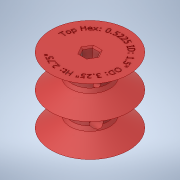
# Autodesk Inventor part: spoolV07
Saved by Autodesk Inventor 2020.2 (Build 242310000, 310)
## iProperties
Created: 2019-02-25
Part Number: spoolV07
Material: PC/ABS Plastic
Document SubType Name: Modeling
Designer: steele
Density: 0.357273 g/cm^3
Appearance: Smooth - Red
holeForString: 0.200 in
stringDiameter: 0.120 in
clearanceForString: 0.080 in
clearanceForHexShaft: 0.023 in
hexDiameter: 0.523 in
supportChannels: 0.150 in
spoolInteriorDiameter: 1.500 in
spoolInteriroRadius: 0.750 in
spoolExteriorDiameter: 3.250 in
spoolExteriorRadius: 1.625 in
spoolFiletRadius: 0.075 in
holeCenter: 0.575 in
hexHoleChamfer: 0.063 in
stringHoleCenterFromHexShaft: 0.361 in
textCircleDiameter: 2.438 in
textHeight: 0.240 in
textDepth: 0.050 in
stringHoleChamfer: 0.188 in
spoolTotalHeight: 3.000 in
spaceHeight: 0.250 in
spacerDiameter: 0.950 in
spoolHeightWithoutSpacer: 2.750 in
Author: steele
Autodesk Inventor part; units mm, degrees
(part 1 of 2)
ref_plane "XZ Plane" through (0, 0, 0) normal (0, 1, 0) x (-1, 0, 0)
ref_plane "XY Plane" through (0, 0, 0) normal (0, 0, 1) x (1, 0, 0)
sketch "Sketch15" plane through (0, 0, 0) normal (0, 0, 1) x (1, 0, 0)
  line L0 (41.275, 0) -> (41.275, 69.85) construction
  line L1 (0, 0) -> (41.275, 0)
  line L2 (0, 69.85) -> (41.275, 69.85)
  line L3 (19.05, 0) -> (19.05, 69.85) construction
  line L4 (0, 69.85) -> (0, 0)
  line L5 (19.05, 17.4625) -> (41.275, 17.4625) construction
  line L6 (41.275, 0) -> (19.05, 12.8316)
  line L7 (41.275, 34.925) -> (19.05, 22.0934)
  line L8 (19.05, 22.0934) -> (41.275, 22.0934) construction
  line L9 (19.05, 22.0934) -> (19.05, 12.8316)
  line L10 (41.275, 34.925) -> (19.05, 47.7566)
  line L11 (19.05, 47.7566) -> (19.05, 57.0184)
  line L12 (19.05, 57.0184) -> (41.275, 69.85)
  line L13 (41.275, 34.925) -> (19.05, 34.925) construction
  line L14 (19.05, 57.0184) -> (41.275, 57.0184) construction
  dimension "d85" = 41.275
  dimension "d86" = 69.85
  dimension "d87" = 19.05
  dimension "d88" = 41.275
  dimension "d89" = 34.925
  dimension "centerLineForSpool" = 17.4625
  dimension "d93" = 30
  dimension "d94" = 30
  dimension "d95" = 30
  dimension "d96" = 30
  constraints: 30 end point, 10 point on line, 3 horizontal, 2 midpoint, 2 perpendicular, 1 collinear, 1 parallel, 1 vertical
  measures "d85" distance from line of L1.start L0
  measures "d86" distance of L0.start L0.end
  measures "d87" distance from line of L3 L1.start
  measures "d88" distance of L2.start L0.end
  measures "d89" distance from line of L7.start L1
  measures "centerLineForSpool" distance from line of L5.start L1
  measures "d93" angle of L6 L1
  measures "d94" angle of L7 L8
  measures "d95" angle of L10 L13
  measures "d96" angle of L12 L14
revolve "Revolution2" add sketch "Sketch15" angle 360 about axis through (0, 69.85, 0) along (0, -1, 0)
sketch "Sketch16" plane through (0, 0, 0) normal (0, -1, 0) x (1, 0, 0)
  line L0 (-7.6623, 0) -> (-3.8312, 6.6357)
  line L1 (-3.8312, 6.6357) -> (3.8312, 6.6357)
  line L2 (3.8312, 6.6357) -> (7.6623, 0)
  line L3 (7.6623, 0) -> (3.8312, -6.6358)
  line L4 (3.8312, -6.6358) -> (-3.8312, -6.6358)
  line L5 (-3.8312, -6.6358) -> (-7.6623, 0)
  point P0 (0, 0)
  point P1 (0, 0)
  dimension "d103" = 13.2715
  constraints: 12 end point, 1 coincident, 1 horizontal, 13 other
  measures "d103" distance between parallel lines of L1 L4
extrude "Extrusion11" cut sketch "Sketch16" against normal through all
sketch "Sketch17" plane through (0, 0, 0) normal (1, 0, 0) x (0, 1, 0)
  circle A0 centre (52.3875, 9.1757) radius 2.54
  circle A1 centre (17.4625, 9.1757) radius 2.54
  line L0 (0, 41.275) -> (0, -41.275) projected
  line L1 (69.85, 41.275) -> (69.85, -41.275) projected
  line L2 (0, 6.6357) -> (69.85, 6.6357) projected
  point P0 (0, 0)
  dimension "d110" = 17.4625
  dimension "d111" = 17.4625
  dimension "d112" = 5.08
  constraints: 2 centre point, 2 tangent, 1 equal radius
  measures "d110" distance from line of A1.centre L0
  measures "d111" distance from line of A0.centre L1
  measures "d112" diameter of A0
extrude "Extrusion13" cut sketch "Sketch17" along normal through all both and the other way through all
ref_plane "Work Plane4" through (-19.05, 0, 0) normal (1, 0, 0) x (0, 1, 0)
sketch "Sketch22" plane through (-19.05, 0, 0) normal (1, 0, 0) x (0, 1, 0)
  spline S0 degree 8 poles (54.9275, 9.1757) (54.9275, 9.4517) (54.8932, 9.7212) (54.8275, 9.9804) (54.7331, 10.2261) (54.613, 10.4557) (54.4698, 10.6669) (54.3066, 10.858) (53.9519, 11.191) (53.76, 11.336) (53.5529, 11.4599) (53.3333, 11.5609) (53.1042, 11.6378) (52.8683, 11.6896) (52.6284, 11.7157) (52.1061, 11.7157) (51.8268, 11.6801) (51.5538, 11.6098) (51.2914, 11.5059) (51.0437, 11.37) (50.815, 11.2041) (50.6094, 11.0111) (50.2522, 10.5794) (50.097, 10.3366) (49.9708, 10.0693) (49.879, 9.7817) (49.8257, 9.479) (49.8146, 9.1672) (49.848, 8.8531) (50.0407, 8.1024) (50.2409, 7.6991) (50.5126, 7.3483) (50.8412, 7.0608) (51.2104, 6.8444) (51.6031, 6.703) (52.001, 6.6357) (52.6651, 6.6357) (52.944, 6.6704) (53.2202, 6.7403) (53.4892, 6.8459) (53.7465, 6.9871) (53.9869, 7.1637) (54.2051, 7.3748) (54.5207, 7.7816) (54.6337, 7.9584) (54.7307, 8.1474) (54.8096, 8.3459) (54.869, 8.5511) (54.9083, 8.76) (54.9275, 8.9692) (54.9275, 9.1757) knots 0 0 0 0 0 0 0 0 0 0.129052 0.129052 0.129052 0.129052 0.129052 0.129052 0.129052 0.253777 0.253777 0.253777 0.253777 0.253777 0.253777 0.253777 0.399469 0.399469 0.399469 0.399469 0.399469 0.399469 0.399469 0.544533 0.544533 0.544533 0.544533 0.544533 0.544533 0.544533 0.751894 0.751894 0.751894 0.751894 0.751894 0.751894 0.751894 0.900801 0.900801 0.900801 0.900801 0.900801 0.900801 0.900801 1 1 1 1 1 1 1 1 1 projected
  circle A0 centre (52.3875, 9.1757) radius 4.7625
  circle A1 centre (52.3875, 9.1757) radius 2.54 construction
  line L0 (52.3875, 6.6357) -> (69.85, 6.6357) construction
  line L1 (69.85, 41.275) -> (69.85, -41.275) construction
  point P0 (0, 0)
  dimension "d121" = 17.4625
  dimension "d122" = 5.08
  dimension "d125" = 9.525
  constraints: 2 centre point, 1 concentric, 1 tangent, 1 vertical alignment
  measures "d121" distance from line of A1.centre L1
  measures "d122" diameter of A1
  measures "d125" diameter of A0
extrude "Extrusion16" cut sketch "Sketch22" along normal blind 11.1125
ref_plane "Work Plane5" through (19.05, 0, 0) normal (1, 0, 0) x (0, 1, 0)
sketch "Sketch23" plane through (19.05, 0, 0) normal (1, 0, 0) x (0, 1, 0)
  line L0 (17.4625, 6.6357) -> (52.3875, 6.6357) projected
  circle A0 centre (17.4625, 9.1757) radius 2.54 construction
  line L1 (0, 41.275) -> (0, -41.275) projected
  circle A1 centre (17.4625, 9.1757) radius 4.7625
  point P0 (0, 0)
  dimension "d127" = 5.08
  dimension "d128" = 17.4625
  dimension "d129" = 9.525
  constraints: 2 centre point, 1 coincident, 1 tangent
  measures "d127" diameter of A0
  measures "d128" distance from line of A0.centre L1
  measures "d129" diameter of A1
extrude "Extrusion17" cut sketch "Sketch23" against normal blind 11.1125
chamfer "Chamfer10" distance 1.5875 angle 45 12 edges at (0, 69.85, -6.6358) (5.7467, 69.85, -3.3179) (5.7467, 69.85, 3.3179) (0, 69.85, 6.6357) (-5.7467, 69.85, 3.3179) (-5.7467, 69.85, -3.3179) (-5.7467, 0, -3.3179) (-5.7467, 0, 3.3179) (0, 0, 6.6357) (5.7467, 0, 3.3179) (5.7467, 0, -3.3179) (0, 0, -6.6358)
chamfer "Chamfer12" distance 2.3813 angle 45 8 edges at (-4.1302, 57.0184, -18.5969) (5.3604, 57.0184, 18.2803) (-4.1302, 47.7566, -18.5969) (5.3604, 47.7566, 18.2803) (-18.2803, 22.0934, -5.3604) (18.5969, 22.0934, 4.1302) (18.5969, 12.8316, 4.1302) (-18.2803, 12.8316, -5.3604)
ref_plane "Work Plane6" through (0, 38.1, 0) normal (0, -1, 0) x (1, 0, 0)
sketch "Sketch24" plane through (0, 69.85, 0) normal (0, 1, 0) x (1, 0, 0)
  circle A0 centre (0, 0) radius 28.575 construction
  line L0 (-28.5166, 1.8645) -> (-33.4283, 2.2505)
  line L1 (-33.4283, 2.2505) -> (-33.5752, 0.3816)
  line L2 (-33.5752, 0.3816) -> (-34.2343, 0.4334)
  line L3 (-34.2343, 0.4334) -> (-33.8823, 4.9117)
  line L4 (-33.8823, 4.9117) -> (-33.2232, 4.8599)
  line L5 (-33.2232, 4.8599) -> (-33.3701, 2.9909)
  line L6 (-33.3701, 2.9909) -> (-28.4584, 2.6048)
  line L7 (-28.4584, 2.6048) -> (-28.5166, 1.8645)
  spline S0 degree 2 poles (-29.4394, 8.8077) (-28.4076, 8.5664) (-27.5153, 7.3113) (-27.7091, 6.4823) knots 0 0 0 1 2 2 2
  spline S1 degree 2 poles (-27.7091, 6.4823) (-27.9081, 5.6313) (-29.2957, 4.9281) (-30.2922, 5.1611) knots 0 0 0 1 2 2 2
  spline S2 degree 2 poles (-30.2922, 5.1611) (-31.3152, 5.4003) (-32.2133, 6.6707) (-32.0215, 7.4908) knots 0 0 0 1 2 2 2
  spline S3 degree 2 poles (-32.0215, 7.4908) (-31.8276, 8.3198) (-30.4668, 9.0479) (-29.4394, 8.8077) knots 0 0 0 1 2 2 2
  spline S4 degree 2 poles (-29.6055, 8.0978) (-30.3991, 8.2834) (-31.3059, 7.8862) (-31.4306, 7.3527) knots 0 0 0 1 2 2 2
  spline S5 degree 2 poles (-31.4306, 7.3527) (-31.5554, 6.8191) (-30.9199, 6.0566) (-30.1262, 5.871) knots 0 0 0 1 2 2 2
  spline S6 degree 2 poles (-30.1262, 5.871) (-29.3546, 5.6906) (-28.4247, 6.087) (-28.3, 6.6205) knots 0 0 0 1 2 2 2
  spline S7 degree 2 poles (-28.3, 6.6205) (-28.1762, 7.1496) (-28.8206, 7.9142) (-29.6055, 8.0978) knots 0 0 0 1 2 2 2
  spline S8 degree 2 poles (-27.9258, 13.0947) (-26.9489, 12.7082) (-26.1634, 11.3211) (-26.445, 10.6095) knots 0 0 0 1 2 2 2
  spline S9 degree 2 poles (-26.445, 10.6095) (-26.5599, 10.3189) (-26.8713, 9.9259) (-27.1019, 9.7493) knots 0 0 0 1 2 2 2
  line L8 (-27.1019, 9.7493) -> (-25.4681, 9.1029)
  line L9 (-25.4681, 9.1029) -> (-25.728, 8.446)
  line L10 (-25.728, 8.446) -> (-31.063, 10.5569)
  line L11 (-31.063, 10.5569) -> (-30.8031, 11.2138)
  line L12 (-30.8031, 11.2138) -> (-30.3947, 11.0522)
  spline S10 degree 2 poles (-30.3947, 11.0522) (-30.5212, 11.3847) (-30.5794, 12.0992) (-30.4411, 12.4487) knots 0 0 0 1 2 2 2
  spline S11 degree 2 poles (-30.4411, 12.4487) (-30.1762, 13.1182) (-28.8185, 13.4479) (-27.9258, 13.0947) knots 0 0 0 1 2 2 2
  spline S12 degree 2 poles (-28.1183, 12.3868) (-28.7878, 12.6517) (-29.6929, 12.518) (-29.8812, 12.0421) knots 0 0 0 1 2 2 2
  spline S13 degree 2 poles (-29.8812, 12.0421) (-29.9912, 11.7642) (-29.9493, 11.1438) (-29.8473, 10.8356) knots 0 0 0 1 2 2 2
  line L13 (-29.8473, 10.8356) -> (-27.6324, 9.9592)
  spline S14 degree 2 poles (-27.6324, 9.9592) (-27.4087, 10.1678) (-27.1711, 10.4975) (-27.0778, 10.7333) knots 0 0 0 1 2 2 2
  spline S15 degree 2 poles (-27.0778, 10.7333) (-26.8762, 11.2428) (-27.4025, 12.1036) (-28.1183, 12.3868) knots 0 0 0 1 2 2 2
  line L14 (-21.978, 18.3743) -> (-22.4128, 17.7722)
  line L15 (-22.4128, 17.7722) -> (-24.6302, 19.3735)
  line L16 (-24.6302, 19.3735) -> (-26.136, 17.2883)
  line L17 (-26.136, 17.2883) -> (-23.9187, 15.687)
  line L18 (-23.9187, 15.687) -> (-24.3535, 15.0849)
  line L19 (-24.3535, 15.0849) -> (-28.8837, 18.3565)
  line L20 (-28.8837, 18.3565) -> (-28.4489, 18.9586)
  line L21 (-28.4489, 18.9586) -> (-26.672, 17.6754)
  line L22 (-26.672, 17.6754) -> (-25.1662, 19.7606)
  line L23 (-25.1662, 19.7606) -> (-26.943, 21.0438)
  line L24 (-26.943, 21.0438) -> (-26.5082, 21.6458)
  line L25 (-26.5082, 21.6458) -> (-21.978, 18.3743)
  spline S16 degree 2 poles (-19.8935, 20.3825) (-20.6053, 19.6726) (-22.1839, 19.6906) (-22.9194, 20.428) knots 0 0 0 1 2 2 2
  spline S17 degree 2 poles (-22.9194, 20.428) (-23.6422, 21.1525) (-23.7394, 22.7697) (-23.1271, 23.3805) knots 0 0 0 1 2 2 2
  spline S18 degree 2 poles (-23.1271, 23.3805) (-22.8513, 23.6555) (-22.265, 23.9206) (-21.9384, 23.9073) knots 0 0 0 1 2 2 2
  spline S19 degree 2 poles (-21.9384, 23.9073) (-21.6086, 23.8973) (-20.9494, 23.5763) (-20.5944, 23.2204) knots 0 0 0 1 2 2 2
  line L26 (-20.5944, 23.2204) -> (-20.3226, 22.9479)
  line L27 (-20.3226, 22.9479) -> (-22.3777, 20.898)
  spline S20 degree 2 poles (-22.3777, 20.898) (-21.8628, 20.3818) (-20.7966, 20.3517) (-20.3349, 20.8122) knots 0 0 0 1 2 2 2
  spline S21 degree 2 poles (-20.3349, 20.8122) (-20.1714, 20.9753) (-19.9275, 21.3656) (-19.8569, 21.5512) knots 0 0 0 1 2 2 2
  spline S22 degree 2 poles (-19.8569, 21.5512) (-19.7862, 21.7497) (-19.7122, 22.0474) (-19.7024, 22.1594) knots 0 0 0 1 2 2 2
  line L28 (-19.7024, 22.1594) -> (-19.6735, 22.1882)
  line L29 (-19.6735, 22.1882) -> (-19.1299, 21.6432)
  spline S23 degree 2 poles (-19.1299, 21.6432) (-19.1813, 21.5216) (-19.3418, 21.1567) (-19.4156, 21.0256) knots 0 0 0 1 2 2 2
  spline S24 degree 2 poles (-19.4156, 21.0256) (-19.5183, 20.84) (-19.714, 20.5616) (-19.8935, 20.3825) knots 0 0 0 1 2 2 2
  spline S25 degree 2 poles (-21.1905, 22.8433) (-21.3984, 23.0389) (-21.776, 23.2507) (-21.9553, 23.2702) knots 0 0 0 1 2 2 2
  spline S26 degree 2 poles (-21.9553, 23.2702) (-22.1537, 23.296) (-22.5446, 23.1428) (-22.7466, 22.9413) knots 0 0 0 1 2 2 2
  spline S27 degree 2 poles (-22.7466, 22.9413) (-22.9453, 22.7431) (-23.1059, 22.3462) (-23.1062, 22.1157) knots 0 0 0 1 2 2 2
  spline S28 degree 2 poles (-23.1062, 22.1157) (-23.1001, 21.8851) (-22.9309, 21.4846) (-22.7582, 21.2795) knots 0 0 0 1 2 2 2
  line L30 (-22.7582, 21.2795) -> (-21.1905, 22.8433)
  line L31 (-15.7374, 23.9237) -> (-16.4275, 23.4023)
  line L32 (-16.4275, 23.4023) -> (-18.1904, 24.0455)
  line L33 (-18.1904, 24.0455) -> (-18.075, 22.1575)
  line L34 (-18.075, 22.1575) -> (-18.7145, 21.6744)
  line L35 (-18.7145, 21.6744) -> (-18.8078, 24.209)
  line L36 (-18.8078, 24.209) -> (-21.2315, 25.0282)
  line L37 (-21.2315, 25.0282) -> (-20.5415, 25.5496)
  line L38 (-20.5415, 25.5496) -> (-18.7903, 24.9146)
  line L39 (-18.7903, 24.9146) -> (-18.9047, 26.7862)
  line L40 (-18.9047, 26.7862) -> (-18.2652, 27.2694)
  line L41 (-18.2652, 27.2694) -> (-18.1703, 24.7474)
  line L42 (-18.1703, 24.7474) -> (-15.7374, 23.9237)
  line L43 (-15.7233, 27.5289) -> (-16.4955, 27.0733)
  line L44 (-16.4955, 27.0733) -> (-17.0386, 27.9937)
  line L45 (-17.0386, 27.9937) -> (-16.2664, 28.4493)
  line L46 (-16.2664, 28.4493) -> (-15.7233, 27.5289)
  line L47 (-14.1354, 24.8379) -> (-14.9076, 24.3823)
  line L48 (-14.9076, 24.3823) -> (-15.4507, 25.3027)
  line L49 (-15.4507, 25.3027) -> (-14.6785, 25.7583)
  line L50 (-14.6785, 25.7583) -> (-14.1354, 24.8379)
  spline S29 degree 2 poles (-8.4241, 30.2696) (-7.9392, 28.8465) (-8.3122, 27.2316) (-9.1738, 26.938) knots 0 0 0 1 2 2 2
  spline S30 degree 2 poles (-9.1738, 26.938) (-10.0482, 26.6401) (-11.3299, 27.7199) (-11.8045, 29.113) knots 0 0 0 1 2 2 2
  spline S31 degree 2 poles (-11.8045, 29.113) (-12.2924, 30.5446) (-11.9164, 32.151) (-11.0505, 32.446) knots 0 0 0 1 2 2 2
  spline S32 degree 2 poles (-11.0505, 32.446) (-10.1804, 32.7425) (-8.8943, 31.6498) (-8.4241, 30.2696) knots 0 0 0 1 2 2 2
  spline S33 degree 2 poles (-8.7836, 28.3483) (-8.7698, 28.6448) (-8.9587, 29.4799) (-9.1442, 30.0242) knots 0 0 0 1 2 2 2
  spline S34 degree 2 poles (-9.1442, 30.0242) (-9.3296, 30.5686) (-9.6885, 31.341) (-9.8877, 31.5745) knots 0 0 0 1 2 2 2
  spline S35 degree 2 poles (-9.8877, 31.5745) (-10.0868, 31.808) (-10.5547, 31.9596) (-10.8504, 31.8588) knots 0 0 0 1 2 2 2
  spline S36 degree 2 poles (-10.8504, 31.8588) (-11.1462, 31.758) (-11.4328, 31.3494) (-11.4493, 31.0328) knots 0 0 0 1 2 2 2
  spline S37 degree 2 poles (-11.4493, 31.0328) (-11.4644, 30.7263) (-11.2612, 29.877) (-11.0844, 29.3584) knots 0 0 0 1 2 2 2
  spline S38 degree 2 poles (-11.0844, 29.3584) (-10.8946, 28.8011) (-10.5719, 28.0787) (-10.3611, 27.8252) knots 0 0 0 1 2 2 2
  spline S39 degree 2 poles (-10.3611, 27.8252) (-10.1648, 27.5859) (-9.6825, 27.4201) (-9.3739, 27.5253) knots 0 0 0 1 2 2 2
  spline S40 degree 2 poles (-9.3739, 27.5253) (-9.0824, 27.6246) (-8.7958, 28.0332) (-8.7836, 28.3483) knots 0 0 0 1 2 2 2
  line L51 (-5.6473, 28.0149) -> (-6.5234, 27.8241)
  line L52 (-6.5234, 27.8241) -> (-6.7508, 28.8683)
  line L53 (-6.7508, 28.8683) -> (-5.8747, 29.0591)
  line L54 (-5.8747, 29.0591) -> (-5.6473, 28.0149)
  spline S41 degree 2 poles (-1.3554, 30.3674) (-1.315, 29.9664) (-1.5028, 29.2556) (-1.7116, 28.9797) knots 0 0 0 1 2 2 2
  spline S42 degree 2 poles (-1.7116, 28.9797) (-1.9205, 28.7038) (-2.5893, 28.3405) (-3.0218, 28.2969) knots 0 0 0 1 2 2 2
  spline S43 degree 2 poles (-3.0218, 28.2969) (-3.4183, 28.2569) (-4.211, 28.3545) (-4.5089, 28.4655) knots 0 0 0 1 2 2 2
  line L55 (-4.5089, 28.4655) -> (-4.5884, 29.254)
  line L56 (-4.5884, 29.254) -> (-4.5343, 29.2594)
  spline S44 degree 2 poles (-4.5343, 29.2594) (-4.4424, 29.205) (-4.1061, 29.075) (-3.9051, 29.0225) knots 0 0 0 1 2 2 2
  spline S45 degree 2 poles (-3.9051, 29.0225) (-3.6766, 28.9681) (-3.303, 28.9193) (-3.0733, 28.9425) knots 0 0 0 1 2 2 2
  spline S46 degree 2 poles (-3.0733, 28.9425) (-2.848, 28.9652) (-2.4408, 29.1701) (-2.3054, 29.3613) knots 0 0 0 1 2 2 2
  spline S47 degree 2 poles (-2.3054, 29.3613) (-2.1825, 29.5421) (-2.0828, 29.9982) (-2.1128, 30.2955) knots 0 0 0 1 2 2 2
  spline S48 degree 2 poles (-2.1128, 30.2955) (-2.1428, 30.5929) (-2.3432, 30.955) (-2.5091, 31.0657) knots 0 0 0 1 2 2 2
  spline S49 degree 2 poles (-2.5091, 31.0657) (-2.6809, 31.1895) (-3.1612, 31.2594) (-3.4451, 31.2307) knots 0 0 0 1 2 2 2
  spline S50 degree 2 poles (-3.4451, 31.2307) (-3.7515, 31.1999) (-4.3502, 31.0439) (-4.5308, 30.9847) knots 0 0 0 1 2 2 2
  line L57 (-4.5308, 30.9847) -> (-4.8198, 33.8502)
  line L58 (-4.8198, 33.8502) -> (-1.7695, 34.1578)
  line L59 (-1.7695, 34.1578) -> (-1.7036, 33.5045)
  line L60 (-1.7036, 33.5045) -> (-4.0375, 33.2692)
  line L61 (-4.0375, 33.2692) -> (-3.888, 31.7869)
  spline S51 degree 2 poles (-3.888, 31.7869) (-3.7547, 31.8185) (-3.4947, 31.8584) (-3.3866, 31.8693) knots 0 0 0 1 2 2 2
  spline S52 degree 2 poles (-3.3866, 31.8693) (-2.9586, 31.9124) (-2.3543, 31.8323) (-2.063, 31.6523) knots 0 0 0 1 2 2 2
  spline S53 degree 2 poles (-2.063, 31.6523) (-1.7673, 31.4728) (-1.4063, 30.872) (-1.3554, 30.3674) knots 0 0 0 1 2 2 2
  line L62 (3.0687, 28.464) -> (-0.3737, 28.6224)
  line L63 (-0.3737, 28.6224) -> (-0.3373, 29.4141)
  spline S54 degree 2 poles (-0.3373, 29.4141) (0.0497, 29.7453) (0.7399, 30.3618) (1.0725, 30.6955) knots 0 0 0 1 2 2 2
  spline S55 degree 2 poles (1.0725, 30.6955) (1.7426, 31.3673) (2.2473, 32.1873) (2.2679, 32.6351) knots 0 0 0 1 2 2 2
  spline S56 degree 2 poles (2.2679, 32.6351) (2.2787, 32.8703) (2.1502, 33.2298) (2.0242, 33.349) knots 0 0 0 1 2 2 2
  spline S57 degree 2 poles (2.0242, 33.349) (1.8982, 33.4681) (1.5596, 33.597) (1.3516, 33.6066) knots 0 0 0 1 2 2 2
  spline S58 degree 2 poles (1.3516, 33.6066) (1.1525, 33.6157) (0.7408, 33.535) (0.5518, 33.4666) knots 0 0 0 1 2 2 2
  spline S59 degree 2 poles (0.5518, 33.4666) (0.3906, 33.4105) (0.0882, 33.2431) (-0.0052, 33.184) knots 0 0 0 1 2 2 2
  line L64 (-0.0052, 33.184) -> (-0.0459, 33.1858)
  line L65 (-0.0459, 33.1858) -> (-0.0092, 33.982)
  spline S60 degree 2 poles (-0.0092, 33.982) (0.2267, 34.0845) (1.0647, 34.268) (1.4356, 34.251) knots 0 0 0 1 2 2 2
  spline S61 degree 2 poles (1.4356, 34.251) (2.2182, 34.2149) (3.0622, 33.3465) (3.0297, 32.6409) knots 0 0 0 1 2 2 2
  spline S62 degree 2 poles (3.0297, 32.6409) (3.0145, 32.3106) (2.8353, 31.7658) (2.6888, 31.5369) knots 0 0 0 1 2 2 2
  spline S63 degree 2 poles (2.6888, 31.5369) (2.5418, 31.2988) (2.1262, 30.8374) (1.8985, 30.6167) knots 0 0 0 1 2 2 2
  spline S64 degree 2 poles (1.8985, 30.6167) (1.5279, 30.2485) (0.6261, 29.4649) (0.3572, 29.237) knots 0 0 0 1 2 2 2
  line L66 (0.3572, 29.237) -> (3.0985, 29.1109)
  line L67 (3.0985, 29.1109) -> (3.0687, 28.464)
  line L68 (7.1904, 27.7113) -> (3.808, 28.3705)
  line L69 (3.808, 28.3705) -> (3.9596, 29.1483)
  spline S65 degree 2 poles (3.9596, 29.1483) (4.3907, 29.4195) (5.1635, 29.9286) (5.5414, 30.2103) knots 0 0 0 1 2 2 2
  spline S66 degree 2 poles (5.5414, 30.2103) (6.3023, 30.7771) (6.9213, 31.5146) (7.007, 31.9546) knots 0 0 0 1 2 2 2
  spline S67 degree 2 poles (7.007, 31.9546) (7.0521, 32.1857) (6.9774, 32.5601) (6.8702, 32.6964) knots 0 0 0 1 2 2 2
  spline S68 degree 2 poles (6.8702, 32.6964) (6.7629, 32.8326) (6.4468, 33.0095) (6.2423, 33.0494) knots 0 0 0 1 2 2 2
  spline S69 degree 2 poles (6.2423, 33.0494) (6.0467, 33.0875) (5.6277, 33.0677) (5.4307, 33.0276) knots 0 0 0 1 2 2 2
  spline S70 degree 2 poles (5.4307, 33.0276) (5.263, 32.9957) (4.9394, 32.8742) (4.8384, 32.8293) knots 0 0 0 1 2 2 2
  line L70 (4.8384, 32.8293) -> (4.7984, 32.8371)
  line L71 (4.7984, 32.8371) -> (4.9509, 33.6194)
  spline S71 degree 2 poles (4.9509, 33.6194) (5.1992, 33.6863) (6.055, 33.7456) (6.4195, 33.6746) knots 0 0 0 1 2 2 2
  spline S72 degree 2 poles (6.4195, 33.6746) (7.1884, 33.5247) (7.8967, 32.5425) (7.7615, 31.8491) knots 0 0 0 1 2 2 2
  spline S73 degree 2 poles (7.7615, 31.8491) (7.6983, 31.5246) (7.4415, 31.0118) (7.2631, 30.8067) knots 0 0 0 1 2 2 2
  spline S74 degree 2 poles (7.2631, 30.8067) (7.083, 30.5926) (6.6045, 30.1968) (6.347, 30.0117) knots 0 0 0 1 2 2 2
  spline S75 degree 2 poles (6.347, 30.0117) (5.9267, 29.7015) (4.9201, 29.058) (4.6208, 28.8718) knots 0 0 0 1 2 2 2
  line L72 (4.6208, 28.8718) -> (7.3143, 28.3469)
  line L73 (7.3143, 28.3469) -> (7.1904, 27.7113)
  spline S76 degree 2 poles (11.6929, 28.0587) (11.5589, 27.6786) (11.0866, 27.1153) (10.7802, 26.9544) knots 0 0 0 1 2 2 2
  spline S77 degree 2 poles (10.7802, 26.9544) (10.4738, 26.7935) (9.714, 26.7493) (9.304, 26.8939) knots 0 0 0 1 2 2 2
  spline S78 degree 2 poles (9.304, 26.8939) (8.9282, 27.0264) (8.2523, 27.4519) (8.0299, 27.6791) knots 0 0 0 1 2 2 2
  line L74 (8.0299, 27.6791) -> (8.2934, 28.4265)
  line L75 (8.2934, 28.4265) -> (8.3447, 28.4085)
  spline S79 degree 2 poles (8.3447, 28.4085) (8.4047, 28.3201) (8.6538, 28.0594) (8.8133, 27.9263) knots 0 0 0 1 2 2 2
  spline S80 degree 2 poles (8.8133, 27.9263) (8.997, 27.7799) (9.3143, 27.5768) (9.5321, 27.5001) knots 0 0 0 1 2 2 2
  spline S81 degree 2 poles (9.5321, 27.5001) (9.7456, 27.4248) (10.2013, 27.437) (10.4052, 27.5524) knots 0 0 0 1 2 2 2
  spline S82 degree 2 poles (10.4052, 27.5524) (10.5933, 27.6637) (10.8775, 28.034) (10.9769, 28.3159) knots 0 0 0 1 2 2 2
  spline S83 degree 2 poles (10.9769, 28.3159) (11.0763, 28.5978) (11.049, 29.0107) (10.946, 29.1815) knots 0 0 0 1 2 2 2
  spline S84 degree 2 poles (10.946, 29.1815) (10.8432, 29.3666) (10.4382, 29.6342) (10.1691, 29.7291) knots 0 0 0 1 2 2 2
  spline S85 degree 2 poles (10.1691, 29.7291) (9.8787, 29.8315) (9.2705, 29.945) (9.0819, 29.9683) knots 0 0 0 1 2 2 2
  line L76 (9.0819, 29.9683) -> (10.0395, 32.6845)
  line L77 (10.0395, 32.6845) -> (12.9308, 31.6652)
  line L78 (12.9308, 31.6652) -> (12.7124, 31.0459)
  line L79 (12.7124, 31.0459) -> (10.5002, 31.8259)
  line L80 (10.5002, 31.8259) -> (10.0049, 30.4208)
  spline S86 degree 2 poles (10.0049, 30.4208) (10.139, 30.3927) (10.3912, 30.3182) (10.4937, 30.282) knots 0 0 0 1 2 2 2
  spline S87 degree 2 poles (10.4937, 30.282) (10.8994, 30.139) (11.4122, 29.8094) (11.5992, 29.5226) knots 0 0 0 1 2 2 2
  spline S88 degree 2 poles (11.5992, 29.5226) (11.7905, 29.2343) (11.8615, 28.537) (11.6929, 28.0587) knots 0 0 0 1 2 2 2
  line L81 (15.7672, 23.8557) -> (13.9176, 24.9801)
  line L82 (13.9176, 24.9801) -> (14.214, 25.4677)
  line L83 (14.214, 25.4677) -> (14.8215, 25.0984)
  line L84 (14.8215, 25.0984) -> (17.1316, 28.8981)
  line L85 (17.1316, 28.8981) -> (16.5241, 29.2674)
  line L86 (16.5241, 29.2674) -> (16.8205, 29.755)
  line L87 (16.8205, 29.755) -> (18.6701, 28.6305)
  line L88 (18.6701, 28.6305) -> (18.3736, 28.143)
  line L89 (18.3736, 28.143) -> (17.7662, 28.5123)
  line L90 (17.7662, 28.5123) -> (15.4561, 24.7126)
  line L91 (15.4561, 24.7126) -> (16.0636, 24.3432)
  line L92 (16.0636, 24.3432) -> (15.7672, 23.8557)
  spline S89 degree 2 poles (21.7285, 22.7421) (21.2429, 22.1506) (19.9819, 21.5921) (19.361, 21.6565) knots 0 0 0 1 2 2 2
  spline S90 degree 2 poles (19.361, 21.6565) (18.8625, 21.72) (18.072, 22.1345) (17.547, 22.5655) knots 0 0 0 1 2 2 2
  line L93 (17.547, 22.5655) -> (16.5529, 23.3815)
  line L94 (16.5529, 23.3815) -> (20.0983, 27.7007)
  line L95 (20.0983, 27.7007) -> (21.0819, 26.8934)
  spline S91 degree 2 poles (21.0819, 26.8934) (21.6909, 26.3935) (22.2346, 25.6426) (22.3474, 25.2805) knots 0 0 0 1 2 2 2
  spline S92 degree 2 poles (22.3474, 25.2805) (22.537, 24.6621) (22.2456, 23.3721) (21.7285, 22.7421) knots 0 0 0 1 2 2 2
  spline S93 degree 2 poles (21.1357, 23.2404) (21.5436, 23.7374) (21.7921, 24.711) (21.6304, 25.1777) knots 0 0 0 1 2 2 2
  spline S94 degree 2 poles (21.6304, 25.1777) (21.5114, 25.5039) (21.0904, 26.0545) (20.7019, 26.3734) knots 0 0 0 1 2 2 2
  line L96 (20.7019, 26.3734) -> (20.2644, 26.7325)
  line L97 (20.2644, 26.7325) -> (17.5349, 23.4073)
  line L98 (17.5349, 23.4073) -> (17.9725, 23.0482)
  spline S95 degree 2 poles (17.9725, 23.0482) (18.354, 22.735) (19.0321, 22.3835) (19.4016, 22.3555) knots 0 0 0 1 2 2 2
  spline S96 degree 2 poles (19.4016, 22.3555) (19.8693, 22.3114) (20.7219, 22.7364) (21.1357, 23.2404) knots 0 0 0 1 2 2 2
  line L99 (23.6053, 21.1625) -> (22.9974, 21.8216)
  line L100 (22.9974, 21.8216) -> (23.783, 22.5462)
  line L101 (23.783, 22.5462) -> (24.3909, 21.8871)
  line L102 (24.3909, 21.8871) -> (23.6053, 21.1625)
  line L103 (21.3086, 19.0441) -> (20.7007, 19.7032)
  line L104 (20.7007, 19.7032) -> (21.4862, 20.4277)
  line L105 (21.4862, 20.4277) -> (22.0941, 19.7686)
  line L106 (22.0941, 19.7686) -> (21.3086, 19.0441)
  line L107 (25.2635, 13.4338) -> (23.8611, 15.7715)
  line L108 (23.8611, 15.7715) -> (24.3504, 16.065)
  line L109 (24.3504, 16.065) -> (24.8722, 15.1952)
  line L110 (24.8722, 15.1952) -> (28.0836, 17.1217)
  line L111 (28.0836, 17.1217) -> (27.5618, 17.9915)
  line L112 (27.5618, 17.9915) -> (28.0006, 18.2547)
  spline S97 degree 2 poles (28.0006, 18.2547) (28.2965, 17.7616) (28.8556, 17.4633) (29.2626, 17.6652) knots 0 0 0 1 2 2 2
  line L113 (29.2626, 17.6652) -> (29.5608, 17.1681)
  line L114 (29.5608, 17.1681) -> (25.2426, 14.5777)
  line L115 (25.2426, 14.5777) -> (25.7528, 13.7273)
  line L116 (25.7528, 13.7273) -> (25.2635, 13.4338)
  line L117 (26.2001, 11.4142) -> (25.8292, 12.2306)
  line L118 (25.8292, 12.2306) -> (26.8022, 12.6726)
  line L119 (26.8022, 12.6726) -> (27.1731, 11.8562)
  line L120 (27.1731, 11.8562) -> (26.2001, 11.4142)
  spline S98 degree 2 poles (29.4027, 7.7133) (29.0192, 7.5894) (28.2849, 7.6234) (27.9712, 7.7696) knots 0 0 0 1 2 2 2
  spline S99 degree 2 poles (27.9712, 7.7696) (27.6575, 7.9157) (27.1616, 8.4931) (27.028, 8.9068) knots 0 0 0 1 2 2 2
  spline S100 degree 2 poles (27.028, 8.9068) (26.9055, 9.286) (26.8341, 10.0815) (26.88, 10.3961) knots 0 0 0 1 2 2 2
  line L121 (26.88, 10.3961) -> (27.6341, 10.6397)
  line L122 (27.6341, 10.6397) -> (27.6508, 10.588)
  spline S101 degree 2 poles (27.6508, 10.588) (27.617, 10.4866) (27.5607, 10.1305) (27.5516, 9.923) knots 0 0 0 1 2 2 2
  spline S102 degree 2 poles (27.5516, 9.923) (27.5465, 9.6882) (27.5774, 9.3127) (27.6484, 9.0929) knots 0 0 0 1 2 2 2
  spline S103 degree 2 poles (27.6484, 9.0929) (27.718, 8.8775) (28.004, 8.5225) (28.2193, 8.4303) knots 0 0 0 1 2 2 2
  spline S104 degree 2 poles (28.2193, 8.4303) (28.4219, 8.3482) (28.8888, 8.3467) (29.1732, 8.4386) knots 0 0 0 1 2 2 2
  spline S105 degree 2 poles (29.1732, 8.4386) (29.4576, 8.5305) (29.7694, 8.8025) (29.8427, 8.988) knots 0 0 0 1 2 2 2
  spline S106 degree 2 poles (29.8427, 8.988) (29.9276, 9.182) (29.8949, 9.6663) (29.8072, 9.9378) knots 0 0 0 1 2 2 2
  spline S107 degree 2 poles (29.8072, 9.9378) (29.7125, 10.2308) (29.4341, 10.7833) (29.3383, 10.9475) knots 0 0 0 1 2 2 2
  line L123 (29.3383, 10.9475) -> (32.0789, 11.8327)
  line L124 (32.0789, 11.8327) -> (33.0212, 8.9155)
  line L125 (33.0212, 8.9155) -> (32.3964, 8.7136)
  line L126 (32.3964, 8.7136) -> (31.6754, 10.9458)
  line L127 (31.6754, 10.9458) -> (30.2577, 10.4878)
  spline S108 degree 2 poles (30.2577, 10.4878) (30.3167, 10.3641) (30.4103, 10.1183) (30.4437, 10.0149) knots 0 0 0 1 2 2 2
  spline S109 degree 2 poles (30.4437, 10.0149) (30.576, 9.6056) (30.6247, 8.9979) (30.51, 8.6753) knots 0 0 0 1 2 2 2
  spline S110 degree 2 poles (30.51, 8.6753) (30.3967, 8.3484) (29.8853, 7.8692) (29.4027, 7.7133) knots 0 0 0 1 2 2 2
  line L128 (33.7683, 6.6315) -> (31.6019, 6.3913)
  line L129 (31.6019, 6.3913) -> (31.511, 6.8764)
  line L130 (31.511, 6.8764) -> (33.6173, 7.4371)
  line L131 (33.6173, 7.4371) -> (33.7683, 6.6315)
  line L132 (34.0286, 5.2428) -> (31.8622, 5.0026)
  line L133 (31.8622, 5.0026) -> (31.7713, 5.4877)
  line L134 (31.7713, 5.4877) -> (33.8776, 6.0484)
  line L135 (33.8776, 6.0484) -> (34.0286, 5.2428)
  spline S111 degree 2 poles (33.4015, -3.3875) (33.0155, -3.6865) (31.9132, -3.9878) (31.2166, -3.9548) knots 0 0 0 1 2 2 2
  spline S112 degree 2 poles (31.2166, -3.9548) (30.5381, -3.9225) (29.4553, -3.5266) (29.0998, -3.1833) knots 0 0 0 1 2 2 2
  spline S113 degree 2 poles (29.0998, -3.1833) (28.7271, -2.8211) (28.3994, -1.8943) (28.4254, -1.347) knots 0 0 0 1 2 2 2
  spline S114 degree 2 poles (28.4254, -1.347) (28.4522, -0.7816) (28.8796, 0.1048) (29.2707, 0.4172) knots 0 0 0 1 2 2 2
  spline S115 degree 2 poles (29.2707, 0.4172) (29.6569, 0.7207) (30.7633, 1.0128) (31.4508, 0.9801) knots 0 0 0 1 2 2 2
  spline S116 degree 2 poles (31.4508, 0.9801) (32.1519, 0.9469) (33.2029, 0.5479) (33.5721, 0.2085) knots 0 0 0 1 2 2 2
  spline S117 degree 2 poles (33.5721, 0.2085) (33.9276, -0.1348) (34.2689, -1.0622) (34.2423, -1.6231) knots 0 0 0 1 2 2 2
  spline S118 degree 2 poles (34.2423, -1.6231) (34.2152, -2.193) (33.7738, -3.0878) (33.4015, -3.3875) knots 0 0 0 1 2 2 2
  spline S119 degree 2 poles (31.2533, -3.1813) (31.8052, -3.2075) (32.6714, -3.0083) (32.9622, -2.8045) knots 0 0 0 1 2 2 2
  spline S120 degree 2 poles (32.9622, -2.8045) (33.2622, -2.5966) (33.5813, -1.9861) (33.5998, -1.5971) knots 0 0 0 1 2 2 2
  spline S121 degree 2 poles (33.5998, -1.5971) (33.6189, -1.1946) (33.3672, -0.5751) (33.0796, -0.3303) knots 0 0 0 1 2 2 2
  spline S122 degree 2 poles (33.0796, -0.3303) (32.8052, -0.0951) (31.9569, 0.1809) (31.4141, 0.2067) knots 0 0 0 1 2 2 2
  spline S123 degree 2 poles (31.4141, 0.2067) (30.315, 0.2588) (29.1042, -0.6085) (29.0675, -1.382) knots 0 0 0 1 2 2 2
  spline S124 degree 2 poles (29.0675, -1.382) (29.0307, -2.1555) (30.1542, -3.1291) (31.2533, -3.1813) knots 0 0 0 1 2 2 2
  spline S125 degree 2 poles (29.9682, -9.5518) (29.2236, -9.3749) (28.1686, -8.4867) (27.9542, -7.9004) knots 0 0 0 1 2 2 2
  spline S126 degree 2 poles (27.9542, -7.9004) (27.7926, -7.4245) (27.8184, -6.5324) (27.9754, -5.8715) knots 0 0 0 1 2 2 2
  line L136 (27.9754, -5.8715) -> (28.2727, -4.6203)
  line L137 (28.2727, -4.6203) -> (33.7094, -5.9119)
  line L138 (33.7094, -5.9119) -> (33.4152, -7.15)
  spline S127 degree 2 poles (33.4152, -7.15) (33.2331, -7.9166) (32.7968, -8.7345) (32.5208, -8.9947) knots 0 0 0 1 2 2 2
  spline S128 degree 2 poles (32.5208, -8.9947) (32.0482, -9.4363) (30.7612, -9.7403) (29.9682, -9.5518) knots 0 0 0 1 2 2 2
  spline S129 degree 2 poles (30.156, -8.8006) (30.7816, -8.9492) (31.7655, -8.7454) (32.114, -8.3954) knots 0 0 0 1 2 2 2
  spline S130 degree 2 poles (32.114, -8.3954) (32.3549, -8.1454) (32.6651, -7.5256) (32.7812, -7.0366) knots 0 0 0 1 2 2 2
  line L139 (32.7812, -7.0366) -> (32.9121, -6.4859)
  line L140 (32.9121, -6.4859) -> (28.7266, -5.4915)
  line L141 (28.7266, -5.4915) -> (28.5958, -6.0422)
  spline S131 degree 2 poles (28.5958, -6.0422) (28.4817, -6.5224) (28.4632, -7.286) (28.6001, -7.6304) knots 0 0 0 1 2 2 2
  spline S132 degree 2 poles (28.6001, -7.6304) (28.7657, -8.07) (29.5215, -8.6498) (30.156, -8.8006) knots 0 0 0 1 2 2 2
  line L142 (26.4607, -10.7965) -> (26.7863, -9.9611)
  line L143 (26.7863, -9.9611) -> (27.782, -10.3493)
  line L144 (27.782, -10.3493) -> (27.4564, -11.1847)
  line L145 (27.4564, -11.1847) -> (26.4607, -10.7965)
  line L146 (29.3719, -11.9314) -> (29.6975, -11.096)
  line L147 (29.6975, -11.096) -> (30.6932, -11.4842)
  line L148 (30.6932, -11.4842) -> (30.3676, -12.3195)
  line L149 (30.3676, -12.3195) -> (29.3719, -11.9314)
  spline S133 degree 2 poles (28.2977, -18.1786) (28.4088, -18.0077) (28.5449, -17.6155) (28.5865, -17.4103) knots 0 0 0 1 2 2 2
  spline S134 degree 2 poles (28.5865, -17.4103) (28.6207, -17.2165) (28.6296, -16.9037) (28.6256, -16.7768) knots 0 0 0 1 2 2 2
  line L150 (28.6256, -16.7768) -> (28.6503, -16.7389)
  line L151 (28.6503, -16.7389) -> (29.3147, -17.1708)
  spline S135 degree 2 poles (29.3147, -17.1708) (29.2916, -17.4474) (29.0134, -18.2658) (28.8086, -18.5809) knots 0 0 0 1 2 2 2
  spline S136 degree 2 poles (28.8086, -18.5809) (28.6013, -18.8998) (28.1637, -19.2905) (27.9011, -19.3953) knots 0 0 0 1 2 2 2
  spline S137 degree 2 poles (27.9011, -19.3953) (27.6198, -19.504) (27.0526, -19.4378) (26.764, -19.2502) knots 0 0 0 1 2 2 2
  spline S138 degree 2 poles (26.764, -19.2502) (26.3767, -18.9985) (26.1228, -18.1096) (26.2788, -17.7034) knots 0 0 0 1 2 2 2
  line L152 (26.2788, -17.7034) -> (26.2333, -17.6738)
  spline S139 degree 2 poles (26.2333, -17.6738) (26.1066, -17.8021) (25.7503, -18.0511) (25.5198, -18.1066) knots 0 0 0 1 2 2 2
  spline S140 degree 2 poles (25.5198, -18.1066) (25.2932, -18.1645) (24.7495, -18.0703) (24.4419, -17.8704) knots 0 0 0 1 2 2 2
  spline S141 degree 2 poles (24.4419, -17.8704) (24.1268, -17.6655) (23.7321, -17.1011) (23.6555, -16.7704) knots 0 0 0 1 2 2 2
  spline S142 degree 2 poles (23.6555, -16.7704) (23.5761, -16.4272) (23.7335, -15.7032) (23.9729, -15.3349) knots 0 0 0 1 2 2 2
  spline S143 degree 2 poles (23.9729, -15.3349) (24.2024, -14.9818) (24.8225, -14.4018) (25.0932, -14.243) knots 0 0 0 1 2 2 2
  line L153 (25.0932, -14.243) -> (25.7576, -14.6749)
  line L154 (25.7576, -14.6749) -> (25.728, -14.7204)
  spline S144 degree 2 poles (25.728, -14.7204) (25.4554, -14.8241) (24.7552, -15.3195) (24.5405, -15.6498) knots 0 0 0 1 2 2 2
  spline S145 degree 2 poles (24.5405, -15.6498) (24.4147, -15.8435) (24.2844, -16.3097) (24.341, -16.5301) knots 0 0 0 1 2 2 2
  spline S146 degree 2 poles (24.341, -16.5301) (24.4, -16.7467) (24.6477, -17.0968) (24.9021, -17.2622) knots 0 0 0 1 2 2 2
  spline S147 degree 2 poles (24.9021, -17.2622) (25.1565, -17.4275) (25.5831, -17.4942) (25.7644, -17.423) knots 0 0 0 1 2 2 2
  spline S148 degree 2 poles (25.7644, -17.423) (25.9457, -17.3518) (26.2523, -17.038) (26.3905, -16.8254) knots 0 0 0 1 2 2 2
  line L155 (26.3905, -16.8254) -> (26.5632, -16.5596)
  line L156 (26.5632, -16.5596) -> (27.0834, -16.8977)
  line L157 (27.0834, -16.8977) -> (26.9476, -17.1065)
  spline S149 degree 2 poles (26.9476, -17.1065) (26.6737, -17.528) (26.7306, -18.3211) (27.1141, -18.5704) knots 0 0 0 1 2 2 2
  spline S150 degree 2 poles (27.1141, -18.5704) (27.2925, -18.6864) (27.6358, -18.7151) (27.7833, -18.6543) knots 0 0 0 1 2 2 2
  spline S151 degree 2 poles (27.7833, -18.6543) (27.9395, -18.5885) (28.1916, -18.3419) (28.2977, -18.1786) knots 0 0 0 1 2 2 2
  line L158 (21.7494, -18.5389) -> (22.3204, -17.8476)
  line L159 (22.3204, -17.8476) -> (23.1444, -18.5282)
  line L160 (23.1444, -18.5282) -> (22.5734, -19.2195)
  line L161 (22.5734, -19.2195) -> (21.7494, -18.5389)
  line L162 (18.5545, -21.8025) -> (21.0369, -19.4122)
  line L163 (21.0369, -19.4122) -> (21.5865, -19.9831)
  spline S152 degree 2 poles (21.5865, -19.9831) (21.5609, -20.4918) (21.5338, -21.4168) (21.5473, -21.8879) knots 0 0 0 1 2 2 2
  spline S153 degree 2 poles (21.5473, -21.8879) (21.5742, -22.8364) (21.8225, -23.7666) (22.1334, -24.0895) knots 0 0 0 1 2 2 2
  spline S154 degree 2 poles (22.1334, -24.0895) (22.2968, -24.2592) (22.6461, -24.4131) (22.8193, -24.4035) knots 0 0 0 1 2 2 2
  spline S155 degree 2 poles (22.8193, -24.4035) (22.9924, -24.394) (23.3188, -24.2368) (23.4689, -24.0924) knots 0 0 0 1 2 2 2
  spline S156 degree 2 poles (23.4689, -24.0924) (23.6124, -23.9542) (23.8369, -23.5997) (23.9172, -23.4155) knots 0 0 0 1 2 2 2
  spline S157 degree 2 poles (23.9172, -23.4155) (23.9874, -23.2599) (24.0738, -22.9252) (24.0951, -22.8167) knots 0 0 0 1 2 2 2
  line L164 (24.0951, -22.8167) -> (24.1244, -22.7885)
  line L165 (24.1244, -22.7885) -> (24.6772, -23.3626)
  spline S158 degree 2 poles (24.6772, -23.3626) (24.5894, -23.6043) (24.1464, -24.3389) (23.8789, -24.5965) knots 0 0 0 1 2 2 2
  spline S159 degree 2 poles (23.8789, -24.5965) (23.3145, -25.1399) (22.1037, -25.1554) (21.6137, -24.6466) knots 0 0 0 1 2 2 2
  spline S160 degree 2 poles (21.6137, -24.6466) (21.3844, -24.4084) (21.1121, -23.9037) (21.0466, -23.6398) knots 0 0 0 1 2 2 2
  spline S161 degree 2 poles (21.0466, -23.6398) (20.9749, -23.3695) (20.9257, -22.7504) (20.9221, -22.4333) knots 0 0 0 1 2 2 2
  spline S162 degree 2 poles (20.9221, -22.4333) (20.9096, -21.911) (20.961, -20.7174) (20.9804, -20.3655) knots 0 0 0 1 2 2 2
  line L166 (20.9804, -20.3655) -> (19.0037, -22.2689)
  line L167 (19.0037, -22.2689) -> (18.5545, -21.8025)
  spline S163 degree 2 poles (16.2528, -25.6877) (16.0187, -25.3597) (15.8288, -24.6495) (15.8731, -24.3063) knots 0 0 0 1 2 2 2
  spline S164 degree 2 poles (15.8731, -24.3063) (15.9174, -23.9631) (16.3176, -23.3157) (16.6714, -23.0631) knots 0 0 0 1 2 2 2
  spline S165 degree 2 poles (16.6714, -23.0631) (16.9957, -22.8316) (17.7323, -22.5227) (18.046, -22.4712) knots 0 0 0 1 2 2 2
  line L168 (18.046, -22.4712) -> (18.5065, -23.1162)
  line L169 (18.5065, -23.1162) -> (18.4623, -23.1478)
  spline S166 degree 2 poles (18.4623, -23.1478) (18.3554, -23.1462) (17.999, -23.2003) (17.7984, -23.2545) knots 0 0 0 1 2 2 2
  spline S167 degree 2 poles (17.7984, -23.2545) (17.5731, -23.3207) (17.2246, -23.4638) (17.0366, -23.598) knots 0 0 0 1 2 2 2
  spline S168 degree 2 poles (17.0366, -23.598) (16.8524, -23.7296) (16.6006, -24.1096) (16.5779, -24.3428) knots 0 0 0 1 2 2 2
  spline S169 degree 2 poles (16.5779, -24.3428) (16.5611, -24.5607) (16.701, -25.0061) (16.8746, -25.2494) knots 0 0 0 1 2 2 2
  spline S170 degree 2 poles (16.8746, -25.2494) (17.0483, -25.4926) (17.402, -25.7075) (17.601, -25.7212) knots 0 0 0 1 2 2 2
  spline S171 degree 2 poles (17.601, -25.7212) (17.8115, -25.7433) (18.2632, -25.5655) (18.4954, -25.3998) knots 0 0 0 1 2 2 2
  spline S172 degree 2 poles (18.4954, -25.3998) (18.746, -25.2208) (19.1883, -24.7882) (19.3157, -24.6472) knots 0 0 0 1 2 2 2
  line L170 (19.3157, -24.6472) -> (20.9892, -26.9912)
  line L171 (20.9892, -26.9912) -> (18.4941, -28.7725)
  line L172 (18.4941, -28.7725) -> (18.1126, -28.2381)
  line L173 (18.1126, -28.2381) -> (20.0217, -26.8751)
  line L174 (20.0217, -26.8751) -> (19.156, -25.6626)
  spline S173 degree 2 poles (19.156, -25.6626) (19.056, -25.7563) (18.8501, -25.9199) (18.7616, -25.9831) knots 0 0 0 1 2 2 2
  spline S174 degree 2 poles (18.7616, -25.9831) (18.4115, -26.2331) (17.8472, -26.4635) (17.505, -26.4518) knots 0 0 0 1 2 2 2
  spline S175 degree 2 poles (17.505, -26.4518) (17.1591, -26.4428) (16.5475, -26.1005) (16.2528, -25.6877) knots 0 0 0 1 2 2 2
  line L175 (16.5435, -30.176) -> (15.6587, -28.1839)
  line L176 (15.6587, -28.1839) -> (16.0935, -27.9504)
  line L177 (16.0935, -27.9504) -> (17.2656, -29.7882)
  line L178 (17.2656, -29.7882) -> (16.5435, -30.176)
  line L179 (15.2988, -30.8445) -> (14.414, -28.8524)
  line L180 (14.414, -28.8524) -> (14.8488, -28.6189)
  line L181 (14.8488, -28.6189) -> (16.0209, -30.4567)
  line L182 (16.0209, -30.4567) -> (15.2988, -30.8445)
  line L183 (5.511, -28.1118) -> (6.2279, -27.9177)
  line L184 (6.2279, -27.9177) -> (6.9428, -30.5577)
  line L185 (6.9428, -30.5577) -> (9.4255, -29.8854)
  line L186 (9.4255, -29.8854) -> (8.7106, -27.2454)
  line L187 (8.7106, -27.2454) -> (9.4274, -27.0513)
  line L188 (9.4274, -27.0513) -> (10.888, -32.445)
  line L189 (10.888, -32.445) -> (10.1712, -32.6391)
  line L190 (10.1712, -32.6391) -> (9.5983, -30.5236)
  line L191 (9.5983, -30.5236) -> (7.1156, -31.1959)
  line L192 (7.1156, -31.1959) -> (7.6885, -33.3114)
  line L193 (7.6885, -33.3114) -> (6.9717, -33.5056)
  line L194 (6.9717, -33.5056) -> (5.511, -28.1118)
  spline S176 degree 2 poles (3.174, -28.3205) (3.7443, -28.2465) (4.4709, -28.8144) (4.5623, -29.5195) knots 0 0 0 1 2 2 2
  line L195 (4.5623, -29.5195) -> (4.861, -31.8232)
  line L196 (4.861, -31.8232) -> (5.3325, -31.7621)
  line L197 (5.3325, -31.7621) -> (5.4076, -32.3414)
  line L198 (5.4076, -32.3414) -> (4.9361, -32.4026)
  line L199 (4.9361, -32.4026) -> (5.091, -33.5971)
  line L200 (5.091, -33.5971) -> (4.3904, -33.6879)
  line L201 (4.3904, -33.6879) -> (4.2355, -32.4934)
  line L202 (4.2355, -32.4934) -> (2.9467, -32.6605)
  line L203 (2.9467, -32.6605) -> (2.8716, -32.0812)
  line L204 (2.8716, -32.0812) -> (4.1604, -31.9141)
  line L205 (4.1604, -31.9141) -> (3.9037, -29.9336)
  spline S177 degree 2 poles (3.9037, -29.9336) (3.8629, -29.6193) (3.7956, -29.2764) (3.7001, -29.1381) knots 0 0 0 1 2 2 2
  spline S178 degree 2 poles (3.7001, -29.1381) (3.6203, -29.016) (3.3205, -28.9225) (3.078, -28.9539) knots 0 0 0 1 2 2 2
  spline S179 degree 2 poles (3.078, -28.9539) (2.9074, -28.976) (2.6019, -29.1207) (2.5341, -29.1614) knots 0 0 0 1 2 2 2
  line L206 (2.5341, -29.1614) -> (2.4937, -29.1667)
  line L207 (2.4937, -29.1667) -> (2.4122, -28.5379)
  spline S180 degree 2 poles (2.4122, -28.5379) (2.6028, -28.4584) (2.9988, -28.3432) (3.174, -28.3205) knots 0 0 0 1 2 2 2
  line L208 (0.7071, -31.6949) -> (1.6031, -31.6622)
  line L209 (1.6031, -31.6622) -> (1.6421, -32.7302)
  line L210 (1.6421, -32.7302) -> (0.746, -32.7628)
  line L211 (0.746, -32.7628) -> (0.7071, -31.6949)
  line L212 (0.5932, -28.5724) -> (1.4893, -28.5397)
  line L213 (1.4893, -28.5397) -> (1.5282, -29.6077)
  line L214 (1.5282, -29.6077) -> (0.6322, -29.6403)
  line L215 (0.6322, -29.6403) -> (0.5932, -28.5724)
  line L216 (-6.5171, -27.8773) -> (-3.1196, -28.4544)
  line L217 (-3.1196, -28.4544) -> (-3.2523, -29.2356)
  spline S181 degree 2 poles (-3.2523, -29.2356) (-3.6768, -29.5172) (-4.437, -30.0449) (-4.8079, -30.3356) knots 0 0 0 1 2 2 2
  spline S182 degree 2 poles (-4.8079, -30.3356) (-5.555, -30.9207) (-6.1558, -31.673) (-6.2309, -32.1149) knots 0 0 0 1 2 2 2
  spline S183 degree 2 poles (-6.2309, -32.1149) (-6.2703, -32.3471) (-6.1866, -32.7196) (-6.0761, -32.8532) knots 0 0 0 1 2 2 2
  spline S184 degree 2 poles (-6.0761, -32.8532) (-5.9656, -32.9868) (-5.6453, -33.156) (-5.4399, -33.1909) knots 0 0 0 1 2 2 2
  spline S185 degree 2 poles (-5.4399, -33.1909) (-5.2435, -33.2243) (-4.825, -33.1943) (-4.629, -33.1495) knots 0 0 0 1 2 2 2
  spline S186 degree 2 poles (-4.629, -33.1495) (-4.4622, -33.1135) (-4.1417, -32.9842) (-4.0417, -32.9369) knots 0 0 0 1 2 2 2
  line L218 (-4.0417, -32.9369) -> (-4.0016, -32.9437)
  line L219 (-4.0016, -32.9437) -> (-4.135, -33.7295)
  spline S187 degree 2 poles (-4.135, -33.7295) (-4.3817, -33.8024) (-5.2358, -33.8824) (-5.6019, -33.8202) knots 0 0 0 1 2 2 2
  spline S188 degree 2 poles (-5.6019, -33.8202) (-6.3742, -33.689) (-7.106, -32.7242) (-6.9877, -32.0277) knots 0 0 0 1 2 2 2
  spline S189 degree 2 poles (-6.9877, -32.0277) (-6.9324, -31.7018) (-6.6881, -31.183) (-6.5147, -30.9736) knots 0 0 0 1 2 2 2
  spline S190 degree 2 poles (-6.5147, -30.9736) (-6.3399, -30.7552) (-5.8711, -30.348) (-5.6181, -30.1567) knots 0 0 0 1 2 2 2
  spline S191 degree 2 poles (-5.6181, -30.1567) (-5.2054, -29.8363) (-4.2147, -29.1686) (-3.9201, -28.9753) knots 0 0 0 1 2 2 2
  line L220 (-3.9201, -28.9753) -> (-6.6255, -28.5157)
  line L221 (-6.6255, -28.5157) -> (-6.5171, -27.8773)
  line L222 (-8.3832, -27.3212) -> (-7.522, -27.5709)
  line L223 (-7.522, -27.5709) -> (-7.8196, -28.5973)
  line L224 (-7.8196, -28.5973) -> (-8.6808, -28.3477)
  line L225 (-8.6808, -28.3477) -> (-8.3832, -27.3212)
  line L226 (-14.5382, -30.0421) -> (-10.4744, -26.5928)
  line L227 (-10.4744, -26.5928) -> (-9.7391, -26.9003)
  line L228 (-9.7391, -26.9003) -> (-13.9981, -30.4643)
  line L229 (-13.9981, -30.4643) -> (-11.3369, -31.5773)
  line L230 (-11.3369, -31.5773) -> (-11.5903, -32.1831)
  line L231 (-11.5903, -32.1831) -> (-14.8614, -30.815)
  line L232 (-14.8614, -30.815) -> (-14.5382, -30.0421)
  spline S192 degree 2 poles (-17.1264, -25.1137) (-16.9183, -24.7686) (-16.3418, -24.3124) (-16.0092, -24.2169) knots 0 0 0 1 2 2 2
  spline S193 degree 2 poles (-16.0092, -24.2169) (-15.6766, -24.1213) (-14.9236, -24.2317) (-14.5513, -24.4562) knots 0 0 0 1 2 2 2
  spline S194 degree 2 poles (-14.5513, -24.4562) (-14.21, -24.6619) (-13.6342, -25.2154) (-13.4624, -25.4829) knots 0 0 0 1 2 2 2
  line L233 (-13.4624, -25.4829) -> (-13.8716, -26.1615)
  line L234 (-13.8716, -26.1615) -> (-13.9182, -26.1335)
  spline S195 degree 2 poles (-13.9182, -26.1335) (-13.9591, -26.0348) (-14.1503, -25.7291) (-14.2796, -25.5665) knots 0 0 0 1 2 2 2
  spline S196 degree 2 poles (-14.2796, -25.5665) (-14.4299, -25.386) (-14.6995, -25.1229) (-14.8973, -25.0037) knots 0 0 0 1 2 2 2
  spline S197 degree 2 poles (-14.8973, -25.0037) (-15.0912, -24.8868) (-15.5399, -24.8066) (-15.763, -24.8783) knots 0 0 0 1 2 2 2
  spline S198 degree 2 poles (-15.763, -24.8783) (-15.9697, -24.9493) (-16.3229, -25.2545) (-16.4773, -25.5104) knots 0 0 0 1 2 2 2
  spline S199 degree 2 poles (-16.4773, -25.5104) (-16.6316, -25.7664) (-16.6884, -26.1763) (-16.622, -26.3644) knots 0 0 0 1 2 2 2
  spline S200 degree 2 poles (-16.622, -26.3644) (-16.5588, -26.5665) (-16.2163, -26.9105) (-15.972, -27.0578) knots 0 0 0 1 2 2 2
  spline S201 degree 2 poles (-15.972, -27.0578) (-15.7083, -27.2168) (-15.1357, -27.451) (-14.9556, -27.512) knots 0 0 0 1 2 2 2
  line L235 (-14.9556, -27.512) -> (-16.4428, -29.9784)
  line L236 (-16.4428, -29.9784) -> (-19.0682, -28.3953)
  line L237 (-19.0682, -28.3953) -> (-18.7291, -27.833)
  line L238 (-18.7291, -27.833) -> (-16.7204, -29.0443)
  line L239 (-16.7204, -29.0443) -> (-15.951, -27.7684)
  spline S202 degree 2 poles (-15.951, -27.7684) (-16.0767, -27.7138) (-16.3087, -27.5898) (-16.4017, -27.5337) knots 0 0 0 1 2 2 2
  spline S203 degree 2 poles (-16.4017, -27.5337) (-16.7701, -27.3115) (-17.2057, -26.885) (-17.3308, -26.5663) knots 0 0 0 1 2 2 2
  spline S204 degree 2 poles (-17.3308, -26.5663) (-17.4597, -26.2453) (-17.3883, -25.548) (-17.1264, -25.1137) knots 0 0 0 1 2 2 2
  line L240 (-22.2383, -26.2849) -> (-20.7611, -24.6821)
  line L241 (-20.7611, -24.6821) -> (-20.3741, -24.9885)
  line L242 (-20.3741, -24.9885) -> (-21.5957, -26.7937)
  line L243 (-21.5957, -26.7937) -> (-22.2383, -26.2849)
  line L244 (-21.1306, -27.162) -> (-19.6534, -25.5592)
  line L245 (-19.6534, -25.5592) -> (-19.2665, -25.8656)
  line L246 (-19.2665, -25.8656) -> (-20.4881, -27.6708)
  line L247 (-20.4881, -27.6708) -> (-21.1306, -27.162)
  dimension "d142" = 57.15
  constraints: 1 centre point, 1 coincident, 1 other
  measures "d142" diameter of A0
extrude "Extrusion18" cut sketch "Sketch24" against normal blind 1.27